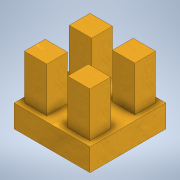
# Autodesk Inventor part: Part27
Saved by Autodesk Inventor 2020 (Build 240168000, 168)
## iProperties
Created: 2021-10-14
Part Number: Part27
Material: Brass, Soft Yellow, Welded
Document SubType Name: Modeling
Designer: simon.erikssonwestl
Density: 8.5 g/cm^3
Appearance: Weld - Brass
Author: simon.erikssonwestl
Autodesk Inventor part; units mm, degrees
ref_plane "YZ Plane" through (0, 0, 0) normal (1, 0, 0) x (0, 1, 0)
ref_plane "XZ Plane" through (0, 0, 0) normal (0, 1, 0) x (-1, 0, 0)
ref_plane "XY Plane" through (0, 0, 0) normal (0, 0, 1) x (1, 0, 0)
sketch "Sketch1" plane through (0, 0, 0) normal (0, 1, 0) x (-1, 0, 0)
  line L0 (5.5, -5.5) -> (-5.5, -5.5)
  line L1 (-5.5, -5.5) -> (-5.5, 5.5)
  line L2 (-5.5, 5.5) -> (5.5, 5.5)
  line L3 (5.5, 5.5) -> (5.5, -5.5)
  line L4 (5.5, -5.5) -> (-5.5, 5.5) construction
  line L5 (-5.5, -5.5) -> (5.5, 5.5) construction
  point P0 (0, 0)
  dimension "d0" = 11
  dimension "d1" = 11
  constraints: 12 end point, 2 midpoint, 2 parallel, 1 horizontal, 1 perpendicular
  measures "d0" distance of L1.end L2.end
  measures "d1" distance of L0.end L1.end
extrude "Extrusion1" add sketch "Sketch1" along normal blind 3.25
sketch "Sketch2" plane through (0, 0, 0) normal (0, -1, 0) x (1, 0, 0)
  line L0 (-4.5, 4.5) -> (4.5, 4.5)
  line L1 (4.5, 4.5) -> (4.5, -4.5)
  line L2 (4.5, -4.5) -> (-4.5, -4.5)
  line L3 (-4.5, -4.5) -> (-4.5, 4.5)
  line L4 (-4.5, 4.5) -> (4.5, -4.5) construction
  line L5 (4.5, 4.5) -> (-4.5, -4.5) construction
  point P0 (0, 0)
  dimension "d4" = 9
  dimension "d5" = 9
  constraints: 12 end point, 2 midpoint, 2 parallel, 1 horizontal, 1 perpendicular
  measures "d4" distance of L1.end L2.end
  measures "d5" distance of L0.end L1.end
extrude "Extrusion2" cut sketch "Sketch2" against normal blind 1
sketch "Sketch3" plane through (0, 3.25, 0) normal (0, 1, 0) x (1, 0, 0)
  line L0 (-4.75, -1.75) -> (-1.5, -1.75)
  line L1 (-1.5, -1.75) -> (-1.5, -4.75)
  line L2 (-1.5, -4.75) -> (-4.75, -4.75)
  line L3 (-4.75, -4.75) -> (-4.75, -1.75)
  line L4 (-4.75, -1.75) -> (-1.5, -4.75) construction
  line L5 (-1.5, -1.75) -> (-4.75, -4.75) construction
  line L6 (-5.5, 5.5) -> (-5.5, -5.5) projected
  line L7 (-5.5, -5.5) -> (5.5, -5.5) projected
  line L8 (-4.75, 4.75) -> (-1.5, 4.75)
  line L9 (-4.75, 1.75) -> (-4.75, 4.75)
  line L10 (-1.5, 4.75) -> (-4.75, 1.75) construction
  line L11 (-1.5, 1.75) -> (-4.75, 1.75)
  line L12 (-1.5, 4.75) -> (-1.5, 1.75)
  line L13 (1.5, -1.75) -> (4.75, -1.75)
  line L14 (1.5, -4.75) -> (1.5, -1.75)
  line L15 (4.75, -1.75) -> (1.5, -4.75) construction
  line L16 (4.75, -4.75) -> (1.5, -4.75)
  line L17 (4.75, -1.75) -> (4.75, -4.75)
  line L18 (1.5, 4.75) -> (4.75, 4.75)
  line L19 (1.5, 1.75) -> (1.5, 4.75)
  line L20 (4.75, 4.75) -> (1.5, 1.75) construction
  line L21 (4.75, 1.75) -> (1.5, 1.75)
  line L22 (4.75, 4.75) -> (4.75, 1.75)
  point P0 (0, 0)
  point P1 (-3.125, -3.25)
  point P2 (-3.125, 3.25)
  point P3 (3.125, -3.25)
  point P4 (3.125, 3.25)
  dimension "d8" = 3.25
  dimension "d9" = 3
  dimension "d10" = 0.75
  dimension "d11" = 0.75
  dimension "d14" = 6.5
  dimension "d17" = 6.25
  constraints: 42 end point, 5 midpoint, 2 horizontal, 2 parallel, 1 perpendicular, 1 vertical, 30 other
  measures "d8" distance of L1.end L2.end
  measures "d9" distance of L0.end L1.end
  measures "d10" distance between parallel lines of L6 L3
  measures "d11" distance between parallel lines of L7 L2
  measures "d14" distance of L0.start L8.start
  measures "d17" distance of L0.start L13.start
extrude "Extrusion3" add sketch "Sketch3" along normal blind 6.5
body "Solid1"
